Top Panel July 13 (Autodesk Fusion 360 design; units mm, degrees)
Autodesk Fusion 360 part; units mm, degrees
sketch "Sketch1" plane through (0, 0, 0) normal (0, 0, 1) x (1, 0, 0)
  line L0 (0, 0) -> (70, 0)
  line L1 (70, 0) -> (70, 240)
  line L2 (70, 240) -> (0, 240)
  line L3 (0, 240) -> (0, 0)
  dimension "d1" = 240
  dimension "d2" = 70
  measures "d1" distance of L0.start L2.end
  measures "d2" distance of L0.start L0.end
extrude "Extrude1" add sketch "Sketch1" along normal blind 2
sketch "Sketch2" plane through (0, 0, 2) normal (0, 0, 1) x (1, 0, 0)
  line L0 (0, 240) -> (0, 0)
  line L1 (0, 0) -> (70, 0)
  line L2 (70, 0) -> (70, 240)
  line L3 (70, 240) -> (0, 240)
  circle A0 centre (40, 50) radius 9
  line L4 (42.958, 41.5) -> (37.042, 41.5)
  line L5 (37.042, 41.5) -> (37.042, 58.5)
  line L6 (37.042, 58.5) -> (42.958, 58.5)
  line L7 (42.958, 58.5) -> (42.958, 41.5)
  circle A1 centre (40, 100) radius 6.25
  line L8 (42.4495, 94.25) -> (37.5505, 94.25)
  line L9 (37.5505, 94.25) -> (37.5505, 105.75)
  line L10 (37.5505, 105.75) -> (42.4495, 105.75)
  line L11 (42.4495, 105.75) -> (42.4495, 94.25)
  point P0 (35, 0)
  point P1 (40, 41.5)
  dimension "d5" = 18
  dimension "d6" = 17
  dimension "d7" = 50
  dimension "d8" = 12.5
  dimension "d9" = 11.5
  dimension "d10" = 50
  dimension "d14" = 40
  measures "d5" diameter of A0
  measures "d6" distance of L4 L6
  measures "d7" distance of A0.centre P0
  measures "d8" diameter of A1
  measures "d9" distance of L8 L10
  measures "d10" distance of A0.centre A1.centre
  measures "d14" distance of L0 A0.centre
extrude "Extrude2" cut sketch "Sketch2" against normal blind 15 contours A0 L7 | L4 L5 L6 L7 | A0 L5 | A1 L11 | L8 L9 L10 L11 | A1 L9
sketch "Sketch3" plane through (0, 0, 2) normal (0, 0, 1) x (1, 0, 0)
  line L0 (42.958, 41.5) -> (37.042, 41.5)
  arc A0 (37.042, 58.5) -> (37.042, 41.5) centre (40, 50) ccw
  line L1 (37.042, 58.5) -> (42.958, 58.5)
  arc A1 (42.958, 41.5) -> (42.958, 58.5) centre (40, 50) ccw
  line L2 (42.4495, 94.25) -> (37.5505, 94.25)
  arc A2 (37.5505, 105.75) -> (37.5505, 94.25) centre (40, 100) ccw
  line L3 (37.5505, 105.75) -> (42.4495, 105.75)
  arc A3 (42.4495, 94.25) -> (42.4495, 105.75) centre (40, 100) ccw
  line L4 (0, 240) -> (0, 0)
  line L5 (0, 0) -> (70, 0)
  line L6 (70, 0) -> (70, 240)
  line L7 (70, 240) -> (0, 240)
  circle A4 centre (7.5, 232.5) radius 1.75
  circle A5 centre (62.5, 232.5) radius 1.75
  circle A6 centre (62.5, 7.5) radius 1.75
  circle A7 centre (7.5, 7.5) radius 1.75
  line L8 (7.5, 232.5) -> (7.5, 7.5) construction
  line L9 (7.5, 7.5) -> (62.5, 7.5) construction
  line L10 (62.5, 7.5) -> (62.5, 232.5) construction
  line L11 (62.5, 232.5) -> (7.5, 232.5) construction
  dimension "d15" = 7.5
  dimension "d16" = 3.5
  dimension "d17" = 3.5
  dimension "d18" = 3.5
  dimension "d19" = 3.5
  measures "d16" diameter of A4
  measures "d17" diameter of A7
  measures "d18" diameter of A6
  measures "d19" diameter of A5
extrude "Extrude3" cut sketch "Sketch3" against normal blind 5 contours A4 | A5 | A6 | A7
sketch "Sketch4" plane through (0, 0, 2) normal (0, 0, 1) x (1, 0, 0)
  circle A0 centre (62.5, 232.5) radius 1.75
  circle A1 centre (7.5, 7.5) radius 1.75
  circle A2 centre (7.5, 232.5) radius 1.75
  circle A3 centre (62.5, 7.5) radius 1.75
  line L0 (42.958, 41.5) -> (37.042, 41.5)
  arc A4 (37.042, 58.5) -> (37.042, 41.5) centre (40, 50) ccw
  line L1 (37.042, 58.5) -> (42.958, 58.5)
  arc A5 (42.958, 41.5) -> (42.958, 58.5) centre (40, 50) ccw
  line L2 (42.4495, 94.25) -> (37.5505, 94.25)
  arc A6 (37.5505, 105.75) -> (37.5505, 94.25) centre (40, 100) ccw
  line L3 (37.5505, 105.75) -> (42.4495, 105.75)
  arc A7 (42.4495, 94.25) -> (42.4495, 105.75) centre (40, 100) ccw
  line L4 (0, 240) -> (0, 0)
  line L5 (0, 0) -> (70, 0)
  line L6 (70, 0) -> (70, 240)
  line L7 (70, 240) -> (0, 240)
  circle A8 centre (22.648, 147.996) radius 1.75
  circle A9 centre (22.648, 180) radius 1.75
  circle A10 centre (45, 147.996) radius 1.75
  circle A11 centre (45, 180) radius 1.75
  dimension "d22" = 3.5
  dimension "d23" = 3.5
  dimension "d24" = 32.004
  dimension "d25" = 3.5
  dimension "d26" = 3.5
  dimension "d27" = 22.352
  dimension "d28" = 25
  dimension "d29" = 60
  measures "d22" diameter of A8
  measures "d23" diameter of A9
  measures "d24" distance of A8.centre A9.centre
  measures "d25" diameter of A10
  measures "d26" diameter of A11
  measures "d27" distance of A8.centre A10.centre
  measures "d28" distance of L6 A10.centre
  measures "d29" distance of L7 A11.centre
extrude "Extrude4" cut sketch "Sketch4" against normal blind 5 contours A8 | A9 | A10 | A11
equation "d1 = 210 mm + 30 mm"
equation "d17 = d16"
equation "d18 = d16"
equation "d19 = d16"
equation "d23 = d22"
equation "d25 = d22"
equation "d26 = d23"
equation "d27 = 1 in - 0.12 in"
